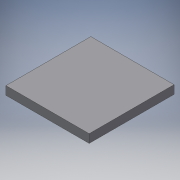
# Autodesk Inventor part: CHAPA_APOIO_INFERIOR_EIXO_X
Saved by Autodesk Inventor 2018 (Build 220112000, 112)
## iProperties
Created: 2018-10-11
Part Number: CHAPA_APOIO_INFERIOR_EIXO_X
Material: Genérico
Document SubType Name: Modeling
Designer: Usuario
Density: 1 g/cm^3
Appearance: Padrão
Author: Usuario
Autodesk Inventor part; units mm, degrees
ref_plane "YZ Plane" through (0, 0, 0) normal (1, 0, 0) x (0, 1, 0)
ref_plane "XZ Plane" through (0, 0, 0) normal (0, 1, 0) x (-1, 0, 0)
ref_plane "XY Plane" through (0, 0, 0) normal (0, 0, 1) x (1, 0, 0)
sketch "Esboço1" plane through (0, 0, 0) normal (0, 0, 1) x (1, 0, 0)
  line L0 (-62.5, 63.75) -> (62.5, 63.75)
  line L1 (62.5, 63.75) -> (62.5, -63.75)
  line L2 (62.5, -63.75) -> (-62.5, -63.75)
  line L3 (-62.5, -63.75) -> (-62.5, 63.75)
  line L4 (-62.5, 63.75) -> (62.5, -63.75) construction
  line L5 (62.5, 63.75) -> (-62.5, -63.75) construction
  point P0 (0, 0)
  dimension "d0" = 125
  dimension "d1" = 127.5
  constraints: 12 end point, 2 midpoint, 2 parallel, 1 horizontal, 1 perpendicular
  measures "d0" distance of L1.end L2.end
  measures "d1" distance of L0.end L1.end
extrude "Extrusão1" add sketch "Esboço1" along normal blind 12.7
